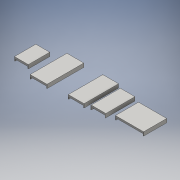
# Autodesk Inventor part: CIRCUIT MOUNT
Saved by Autodesk Inventor 2016 (Build 200138000, 138)
## iProperties
Created: 2017-07-15
Part Number: CIRCUIT MOUNT
Material: Generic
Document SubType Name: Modeling
Designer: ALIREZA
Density: 1 g/cm^3
Appearance: Default
Author: ALIREZA
Autodesk Inventor part; units mm, degrees
ref_plane "YZ Plane" through (0, 0, 0) normal (1, 0, 0) x (0, 1, 0)
ref_plane "XZ Plane" through (0, 0, 0) normal (0, 1, 0) x (-1, 0, 0)
ref_plane "XY Plane" through (0, 0, 0) normal (0, 0, 1) x (1, 0, 0)
sketch "Sketch1" plane through (0, 0, 0) normal (0, 0, 1) x (1, 0, 0)
  point P0 (0, 0)
sketch "Sketch2" plane through (0, 0, 0) normal (0, 0, 1) x (1, 0, 0)
  line L0 (-9.25, -22.217934) -> (-9.25, 23)
  line L1 (-9.25, 23) -> (9.25, 23)
  line L2 (9.25, -23) -> (-9.25, 23) construction
  line L3 (-9.25, -23) -> (9.25, 23) construction
  line L4 (-10, 23.75) -> (10, 23.75)
  line L5 (10, 23.75) -> (10, -22.217934)
  line L6 (-10, -22.217934) -> (-10, 23.75)
  line L7 (-10, 23.75) -> (10, -23.75) construction
  line L8 (10, 23.75) -> (-10, -23.75) construction
  line L9 (-58.307494, 23.75) -> (-37.307494, 23.75)
  line L10 (-37.307494, 23.75) -> (-37.307494, -23.75)
  line L11 (-37.307494, -23.75) -> (-58.307494, -23.75)
  line L12 (-58.307494, -23.75) -> (-58.307494, 23.75)
  line L13 (-58.307494, 23.75) -> (-37.307494, -23.75) construction
  line L14 (-37.307494, 23.75) -> (-58.307494, -23.75) construction
  line L15 (-59.057494, 24.5) -> (-36.557494, 24.5)
  line L16 (-36.557494, 24.5) -> (-36.557494, -24.5)
  line L17 (-36.557494, -24.5) -> (-59.057494, -24.5)
  line L18 (-59.057494, -24.5) -> (-59.057494, 24.5)
  line L19 (-59.057494, 24.5) -> (-36.557494, -24.5) construction
  line L20 (-36.557494, 24.5) -> (-59.057494, -24.5) construction
  line L21 (-89.43439, 13.5) -> (-72.43439, 13.5)
  line L22 (-72.43439, 13.5) -> (-72.43439, -13.5)
  line L23 (-72.43439, -13.5) -> (-89.43439, -13.5)
  line L24 (-89.43439, -13.5) -> (-89.43439, 13.5)
  line L25 (-89.43439, 13.5) -> (-72.43439, -13.5) construction
  line L26 (-72.43439, 13.5) -> (-89.43439, -13.5) construction
  line L27 (-90.18439, -14.25) -> (-90.18439, 14.25)
  line L28 (-90.18439, 14.25) -> (-71.68439, 14.25)
  line L29 (-71.68439, 14.25) -> (-71.68439, -14.25)
  line L30 (-71.68439, -14.25) -> (-90.18439, 14.25) construction
  line L31 (-90.18439, -14.25) -> (-71.68439, 14.25) construction
  line L32 (17.56678, 19) -> (35.56678, 19)
  line L33 (35.56678, 19) -> (35.56678, -19)
  line L34 (35.56678, -19) -> (17.56678, -19)
  line L35 (17.56678, -19) -> (17.56678, 19)
  line L36 (17.56678, 19) -> (35.56678, -19) construction
  line L37 (35.56678, 19) -> (17.56678, -19) construction
  line L38 (16.81678, -19.75) -> (16.81678, 19.75)
  line L39 (16.81678, 19.75) -> (36.31678, 19.75)
  line L40 (36.31678, 19.75) -> (36.31678, -19.75)
  line L41 (36.31678, -19.75) -> (16.81678, 19.75) construction
  line L42 (16.81678, -19.75) -> (36.31678, 19.75) construction
  line L43 (81.776505, -14.991674) -> (81.776505, 15)
  line L44 (81.776505, 15) -> (45.776505, 15)
  line L45 (45.776505, 15) -> (45.776505, -15)
  line L46 (45.776505, -15) -> (81.776505, 15) construction
  line L47 (81.776505, -14.991674) -> (45.776505, 15) construction
  line L48 (45.026505, 15.75) -> (82.526505, 15.75)
  line L49 (82.526505, 15.75) -> (82.526505, -14.974995)
  line L50 (45.026505, -15) -> (45.026505, 15.75)
  line L51 (45.026505, 15.75) -> (82.09375, -15.378222) construction
  line L52 (82.526505, 15.75) -> (63.776505, 0) construction
  line L53 (46.395553, -15) -> (45.526505, -15.75) construction
  line L54 (81.776505, -14.991674) -> (82.526505, -14.974995)
  line L55 (45.776505, -15) -> (45.026505, -15)
  line L56 (-9.25, -23.75) -> (-9.55163, -23.75)
  line L57 (-10, -22.217934) -> (-9.25, -22.217934)
  line L58 (9.25, -22.217934) -> (10, -22.217934)
  line L59 (9.25, 23) -> (9.25, 21.96875)
  line L60 (9.25, -21.96875) -> (9.25, -22.217934)
  line L61 (9.25, -21.96875) -> (9.25, 23)
  line L62 (-89.43439, -13.5) -> (-89.43439, -14.25)
  line L63 (-72.43439, -13.5) -> (-72.43439, -14.25)
  line L64 (-71.68439, -14.25) -> (-72.43439, -14.25)
  line L65 (-89.43439, -14.25) -> (-90.18439, -14.25)
  line L66 (0, 0) -> (0, -5.712725)
  line L67 (17.56678, -19) -> (16.81678, -19.75)
  line L68 (35.56678, -19) -> (36.31678, -19.75)
  line L69 (36.31678, -19.75) -> (35.56678, -19.75)
  line L70 (17.56678, -19.75) -> (16.81678, -19.75)
  line L71 (63.776505, 0) -> (63.776505, -4.283489)
  point P0 (-47.807494, 0)
  point P1 (-47.807494, 0)
  point P2 (-80.93439, 0)
  point P3 (-80.93439, 0)
  point P4 (26.56678, 0)
  point P5 (63.779004, 0.002082)
  dimension "d0" = 18.5
  dimension "d3" = 47.5
  dimension "d4" = 21
  dimension "d5" = 47.5
  dimension "d6" = 22.5
  dimension "d7" = 49
  dimension "d8" = 17
  dimension "d9" = 27
  dimension "d10" = 18.5
  dimension "d11" = 28.5
  dimension "d12" = 18
  dimension "d13" = 38
  dimension "d14" = 19.5
  dimension "d15" = 39.5
  dimension "d16" = 36
  dimension "d24" = 20
  dimension "d25" = 37.5
  constraints: 144 end point, 21 parallel, 20 midpoint, 17 perpendicular, 10 horizontal, 9 point on line, 4 vertical, 5 other
  measures "d0" distance of L0.end L1.end
  measures "d3" distance of L4.end L7.end
  measures "d4" distance of L10.end L11.end
  measures "d5" distance of L9.end L10.end
  measures "d6" distance of L16.end L17.end
  measures "d7" distance of L15.end L16.end
  measures "d8" distance of L22.end L23.end
  measures "d9" distance of L21.end L22.end
  measures "d10" distance of L27.end L28.end
  measures "d11" distance of L27.start L27.end
  measures "d12" distance of L33.end L34.end
  measures "d13" distance of L32.end L33.end
  measures "d14" distance of L38.end L39.end
  measures "d15" distance of L38.start L38.end
  measures "d16" distance of L44.end L43.end
  measures "d24" distance between parallel lines of L5 L6
  measures "d25" distance between parallel lines of L50 L49
extrude "Extrusion1" add sketch "Sketch2" along normal blind 5 contours L57 L6 L4 L5 L58 L60 L61 L59 L1 L0 | L15 L16 L17 L18 | L24 L62 L65 L27 L28 L29 L64 L63 L22 L21 | L35 L67 L38 L39 L40 L68 L33 L32 | L43 L44 L45 L55 L50 L48 L49 L54
sketch "Sketch3" plane through (0, 0, 5) normal (0, 0, 1) x (1, 0, 0)
  line L0 (-9.25, -22.217934) -> (-9.25, 23)
  line L1 (-9.25, 23) -> (9.25, 23)
  line L2 (9.25, 23) -> (9.25, -22.217934)
  line L3 (17.56678, -19) -> (17.56678, 19)
  line L4 (17.56678, 19) -> (35.56678, 19)
  line L5 (35.56678, 19) -> (35.56678, -19)
  line L6 (35.56678, -19) -> (17.56678, -19)
  line L7 (45.776505, -15) -> (45.776505, 15)
  line L8 (45.776505, 15) -> (81.776505, 15)
  line L9 (81.776505, 15) -> (81.776505, -14.991674)
  line L10 (-58.307494, 23.75) -> (-37.307494, 23.75)
  line L11 (-58.307494, -23.75) -> (-58.307494, 23.75)
  line L12 (-37.307494, 23.75) -> (-37.307494, -23.75)
  line L13 (-37.307494, -23.75) -> (-58.307494, -23.75)
  line L14 (-72.43439, 13.5) -> (-72.43439, -14.25)
  line L15 (-89.43439, 13.5) -> (-72.43439, 13.5)
  line L16 (-89.43439, -14.25) -> (-89.43439, 13.5)
  line L17 (9.25, -22.217934) -> (-9.25, -22.217934)
  line L18 (81.776505, -15) -> (45.776505, -15)
  line L19 (-71.68439, -14.25) -> (-71.68439, 14.25)
  line L20 (-89.43439, -14.25) -> (-71.68439, -14.25)
  line L21 (-71.68439, -14.25) -> (-71.68439, 14.25)
  line L22 (-71.68439, 14.25) -> (-90.18439, 14.25)
  line L23 (-90.18439, 14.25) -> (-90.18439, -14.25)
  line L24 (-90.18439, 14.25) -> (-90.18439, -14.25)
  line L25 (-89.43439, -14.25) -> (-89.43439, 13.5)
  line L26 (-90.18439, -14.25) -> (-89.43439, -14.25)
  line L27 (-89.43439, -14.25) -> (-72.43439, -14.25)
  point P0 (0, 0)
  point P1 (-72.43439, -12.5)
  point P2 (-89.43439, -12.5)
  constraints: 14 end point, 2 collinear, 2 horizontal, 1 parallel, 1 perpendicular, 1 vertical
sketch "Sketch3 outline for Extrusion2" plane through (0, 0, 5) normal (0, 0, 1) x (1, 0, 0)
  line L0 (-72.43439, 13.5) -> (-89.43439, 13.5)
  line L1 (-89.43439, 13.5) -> (-89.43439, -14.25)
  line L2 (-89.43439, -14.25) -> (-72.43439, -14.25)
  line L3 (-72.43439, -14.25) -> (-72.43439, 13.5)
  line L4 (17.56678, -19) -> (17.56678, 19)
  line L5 (17.56678, 19) -> (35.56678, 19)
  line L6 (35.56678, 19) -> (35.56678, -19)
  line L7 (35.56678, -19) -> (17.56678, -19)
  line L8 (-58.307494, 23.75) -> (-37.307494, 23.75)
  line L9 (-37.307494, 23.75) -> (-37.307494, -23.75)
  line L10 (-37.307494, -23.75) -> (-58.307494, -23.75)
  line L11 (-58.307494, -23.75) -> (-58.307494, 23.75)
  line L12 (-9.25, -22.217934) -> (-9.25, 23)
  line L13 (-9.25, 23) -> (9.25, 23)
  line L14 (9.25, 23) -> (9.25, -22.217934)
  line L15 (9.25, -22.217934) -> (-9.25, -22.217934)
  line L16 (45.776505, -15) -> (45.776505, 15)
  line L17 (45.776505, 15) -> (81.776505, 15)
  line L18 (81.776505, 15) -> (81.776505, -14.991674)
  line L19 (81.776505, -14.991674) -> (45.776505, -15)
extrude "Extrusion2" add sketch "Sketch3 outline for Extrusion2" against normal blind 2.5
sketch "Sketch4" plane through (0, 0, 0) normal (0, 0, -1) x (-1, 0, 0)
  line L0 (-9.25, -22.217934) -> (9.25, -22.217934)
  line L1 (-9.25, 23) -> (9.25, 23)
  line L2 (9.75, -23) -> (-9.75, -23)
  line L3 (-9.75, -23) -> (-9.75, 23)
  line L4 (-9.75, 23) -> (9.75, 23)
  line L5 (9.75, 23) -> (9.75, -23)
  line L6 (9.75, -23) -> (-9.75, 23) construction
  line L7 (-9.75, -23) -> (9.75, 23) construction
  point P0 (0, 0)
  dimension "d26" = 19.5
  constraints: 12 end point, 2 midpoint, 2 parallel, 1 horizontal, 1 perpendicular, 1 point on line
  measures "d26" distance of L3.end L4.end
extrude "Extrusion3" cut sketch "Sketch4" against normal up to surface (2.5 mm away)
sketch "Sketch5" plane through (0, 0, 0) normal (0, 0, -1) x (-1, 0, 0)
  line L0 (10, 23.75) -> (-10, 23.75)
  line L1 (-10.5, -22.217934) -> (-10.5, 23.75)
  line L2 (-10.5, 23.75) -> (10.5, 23.75)
  line L3 (10.5, 23.75) -> (10.5, -22.217934)
  line L4 (10.5, -23.75) -> (-10.5, 23.75) construction
  line L5 (-10.5, -23.75) -> (10.5, 23.75) construction
  line L6 (-9.75, -22.217934) -> (-9.75, 23)
  line L7 (9.75, 23) -> (9.75, -22.217934)
  line L8 (-9.75, 23) -> (9.75, 23)
  line L9 (9.75, -22.217934) -> (-9.75, -22.217934)
  line L10 (9.75, -22.217934) -> (10.5, -22.217934)
  line L11 (-9.75, -22.217934) -> (-10.5, -22.217934)
  line L12 (10.5, -23.75) -> (9.75, -23.75)
  line L13 (-9.75, -23.75) -> (-10.5, -23.75)
  point P0 (0, 0)
  dimension "d29" = 21
  constraints: 18 end point, 4 point on line, 3 parallel, 3 perpendicular, 2 horizontal, 2 midpoint
  measures "d29" distance of L1.end L2.end
extrude "Extrusion4" add sketch "Sketch5" against normal up to surface (5 mm away) contours L2 L3 L10 L7 L8 L6 L11 L1 L0
sketch "Sketch6" plane through (0, 0, 0) normal (0, 0, -1) x (-1, 0, 0)
  line L0 (58.307494, 23.75) -> (58.307494, -23.75)
  line L1 (58.307494, -22.276606) -> (37.307494, -22.276606)
  line L2 (37.307494, -22.276606) -> (37.307494, -28.128935)
  line L3 (37.307494, -28.128935) -> (58.307494, -28.128935)
  line L4 (58.307494, -28.128935) -> (58.307494, -22.276606)
  point P0 (0, 0)
  constraints: 8 end point, 2 parallel, 1 horizontal, 1 perpendicular, 1 point on line
extrude "Extrusion5" cut sketch "Sketch6" against normal up to surface (2.5 mm away)
body "Solid1"
